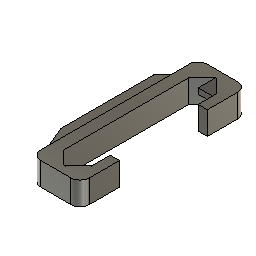
hook big v2 (Autodesk Fusion 360 design; units mm, degrees)
Autodesk Fusion 360 part; units mm, degrees
sketch "Skizze1" plane through (0, 0, 0) normal (0, 0, 1) x (1, 0, 0)
  line L0 (0, 0) -> (6, 0)
  line L1 (6, 29) -> (0, 29)
  line L2 (0, 29) -> (0, 0)
  line L3 (-2.5, 32.5) -> (8, 32.5)
  line L4 (8, -3.5) -> (-2.5, -3.5)
  line L5 (-2.5, -3.5) -> (-2.5, 32.5)
  line L6 (3.6452, 24) -> (13.0618, 24)
  line L7 (3.4597, 5) -> (13.6888, 5)
  line L8 (6, 0) -> (6, 5)
  line L9 (6, 24) -> (6, 29)
  line L10 (8, 32.5) -> (8, 24)
  line L11 (8, 5) -> (8, -3.5)
  dimension "d1" = 29
  dimension "d2" = 6
  dimension "d3" = 2.5
  dimension "d4" = 2
  dimension "d5" = 3.5
  dimension "d6" = 3.5
  dimension "d7" = 5
  dimension "d8" = 5
  constraint horizontal L0
  constraint vertical L8
  constraint horizontal L1
  constraint vertical L2
  constraint coincident L0.start L2.end
  constraint horizontal L3
  constraint vertical L10
  constraint horizontal L4
  constraint vertical L5
  constraint perpendicular L2 L6
  constraint perpendicular L7 L8
  constraint coincident L7 L8.end
  constraint coincident L6 L9.start
  constraint collinear L8 L9
  constraint coincident L6 L10.end
  constraint coincident L7 L11.start
  constraint collinear L10 L11
  measures "d1" distance of L0.start L1.end
  measures "d2" distance of L0.start L0.end
  measures "d3" distance of L2 L5
  measures "d4" distance of L8 L10
  measures "d5" distance of L1 L3
  measures "d6" distance of L0 L4
  measures "d7" distance of L1 L6
  measures "d8" distance of L0 L7
extrude "Extrusion1" add sketch "Skizze1" along normal blind 5
chamfer "Fase1" distance 1 angle 45 4 edges at (0, 29, 2.5) (6, 0, 2.5) (0, 0, 2.5) (6, 29, 2.5)
chamfer "Fase2" distance 1.9 angle 45 4 edges at (3, 29, 5) (3, 0, 5) (3, 0, 0) (3, 29, 0)
fillet "Abrundung1" radius 2 4 edges at (8, 32.5, 2.5) (-2.5, 32.5, 2.5) (-2.5, -3.5, 2.5) (8, -3.5, 2.5)
sketch "Skizze2" plane through (0, 0, 0) normal (0, 0, -1) x (1, 0, 0)
  arc A0 (8, 1.5) -> (6, 3.5) centre (6, 1.5) ccw
  line L0 (6, 3.5) -> (-0.5, 3.5)
  arc A1 (-0.5, 3.5) -> (-2.5, 1.5) centre (-0.5, 1.5) ccw
  line L1 (-2.5, 1.5) -> (-2.5, -30.5)
  arc A2 (-2.5, -30.5) -> (-0.5, -32.5) centre (-0.5, -30.5) ccw
  line L2 (-0.5, -32.5) -> (6, -32.5)
  arc A3 (6, -32.5) -> (8, -30.5) centre (6, -30.5) ccw
  line L3 (8, -30.5) -> (8, -24)
  line L4 (8, -24) -> (6, -24)
  line L5 (6, -24) -> (6, -28)
  line L6 (6, -28) -> (3.1, -30.9)
  line L7 (3.1, -30.9) -> (2.9, -30.9)
  line L8 (2.9, -30.9) -> (0, -28)
  line L9 (0, -28) -> (0, -1)
  line L10 (0, -1) -> (2.9, 1.9)
  line L11 (2.9, 1.9) -> (3.1, 1.9)
  line L12 (3.1, 1.9) -> (6, -1)
  line L13 (6, -1) -> (6, -5)
  line L14 (6, -5) -> (8, -5)
  line L15 (8, -5) -> (8, 1.5)
  line L16 (-2.5, -30.5) -> (-2.5, 1.5)
  line L17 (-2.5, -30.5) -> (-3.5, -30.5)
  line L18 (-3.5, -30.5) -> (-3.5, -11.5)
  line L19 (-3.5, 1.5) -> (-2.5, 1.5)
  line L20 (-2.5, 1.5) -> (-2.5, -30.5)
  line L21 (-4.5, -30.5) -> (-4.5, -11.5)
  line L22 (-4.5, -11.5) -> (-3.5, -11.5)
  line L23 (-3.5, -11.5) -> (-3.5, -30.5)
  line L24 (-4.5, -30.5) -> (-7.3284, -27.6716)
  line L25 (-4.5, -30.5) -> (-0.5, -30.5) construction
  line L26 (-7.3284, -27.6716) -> (-7.3284, -7.6716)
  line L27 (-7.3284, -7.6716) -> (-3.5, 1.5)
  dimension "d14" = 1
  dimension "d15" = 19
  dimension "d16" = 1
  dimension "d17" = 135
  dimension "d18" = 4
  dimension "d19" = 20
  constraint coincident L1.end A2.start
  constraint coincident A1.end L1.start
  constraint horizontal L17
  constraint vertical L18
  constraint horizontal L19
  constraint vertical L20
  constraint vertical L21
  constraint horizontal L22
  constraint vertical L23
  constraint horizontal L25
  constraint vertical L26
  measures "d14" distance of L1.end L17.end
  measures "d15" distance of L17.end L18.end
  measures "d16" distance of L17.end L21.start
  measures "d17" angle of L24 L25
  measures "d18" distance of L21.start L24.end
  measures "d19" distance of L24.end L26.end
extrude "Extrusion2" add sketch "Skizze2" against normal blind 2 contours L1 L16 L17 L18 L19 L20 L21 L22 L23 L24 L26 L27
chamfer "Fase3" distance 1 angle 45 1 edges at (-3.5, -1.5, 1)
chamfer "Fase4" distance 1 angle 45 1 edges at (-2.5, 14.5, 2)
chamfer "Fase5" distance 1 angle 45 1 edges at (-2.5, 30.5, 1.5)
equation "d8 = d7"
